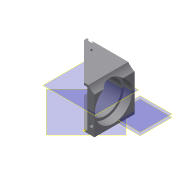
# Autodesk Inventor part: 30_Cube_Insert_Filter_Revolver_Filter_base
Saved by Autodesk Inventor 2019.4 (Build 234330000, 330)
## iProperties
Created: 2021-09-13
Part Number: 30_Cube_Insert_Filter_Revolver_Filter_base
Material: Generic
Document SubType Name: Modeling
Designer: diederichbenedict
Density: 1 g/cm^3
Appearance: Default
Mass: 6.97028 g
Surface Area: 48.8121 cm^2
Volume: 6.97028 cm^3
Author: diederichbenedict
Autodesk Inventor part; units mm, degrees
ref_plane "YZ Plane" through (0, 0, 0) normal (1, 0, 0) x (0, 1, 0)
ref_plane "XZ Plane" through (0, 0, 0) normal (0, 1, 0) x (-1, 0, 0)
ref_plane "XY Plane" through (0, 0, 0) normal (0, 0, 1) x (1, 0, 0)
ref_plane "Work Plane1" through (-34.3358, -34.38, 2.0699) normal (0, -1, 0) x (0.7071068, 0, -0.7071068)
ref_plane "Work Plane4" through (-9.5871, -34.38, 28.2329) normal (0, -1, 0) x (1, 0, 0)
ref_plane "Work Plane3" through (-9.5871, -32.38, 28.2329) normal (0, -1, 0) x (1, 0, 0)
sketch "Sketch1" plane through (-9.5871, -34.38, 28.2329) normal (0, -1, 0) x (1, 0, 0)
  line L0 (-24.2504, -24.2504) -> (-24.2504, -25.6646) construction
  line L1 (-24.2504, -25.6646) -> (0.7071, -0.7071) construction
  line L2 (0.7071, -0.7071) -> (0, 0) construction
  line L3 (-24.2504, -24.2504) -> (0, 0) construction
  line L4 (0.7071, -1.3185) -> (0.7071, -26.3185) construction
  line L5 (0.7071, -1.3185) -> (1.7071, -1.3185) construction
  line L6 (0.7071, -26.3185) -> (1.7071, -26.3185) construction
  line L7 (0.7071, -0.7071) -> (-26.8187, -28.2329)
  line L8 (-26.8187, -28.2329) -> (0.7071, -28.2329)
  line L9 (0.7071, -28.2329) -> (0.7071, -0.7071)
  line L10 (0.7071, -0.7071) -> (5.7071, -0.7071)
  line L11 (5.7071, -0.7071) -> (5.7071, -28.2329)
  line L12 (5.7071, -28.2329) -> (0.7071, -28.2329)
  line L13 (-38.6685, -28.2329) -> (-7.1719, -28.2329) projected
  line L14 (0.7071, -0.7071) -> (5.7071, -0.7071)
  line L15 (5.7071, -0.7071) -> (5.7071, 1.3671)
  line L16 (5.7071, 1.3671) -> (0.7071, 1.3671)
  line L17 (0.7071, 1.3671) -> (0.7071, -0.7071)
  line L18 (2.5336, 1.8671) -> (2.3871, 1.8671) projected
  line L19 (0.7071, -0.7071) -> (0.7071, -28.2329)
  line L20 (0.7071, -28.2329) -> (-26.8187, -28.2329)
  line L21 (-26.8187, -28.2329) -> (0.7071, -0.7071)
  point P0 (9.5871, -28.2329)
  dimension "d1" = 5
  dimension "d2" = 0
  dimension "d3" = 0.5
  constraints: 30 end point, 5 perpendicular, 3 equal length, 3 horizontal, 2 point on line, 2 other
  measures "d1" distance of L9.end L10.end
  measures "d2" distance between parallel lines of L13 L8
  measures "d3" distance between parallel lines of L16 L18
extrude "Extrusion1" add sketch "Sketch1" against normal blind 29 contours L9 L8 L7 | L10 L11 L12 L9
sketch "Sketch2" plane through (-8.88, -34.38, 27.5258) normal (-0.7071068, 0, 0.7071068) x (0.7071068, 0, 0.7071068)
  line L0 (-38.9273, 0) -> (0, 0) projected
  line L1 (0, 0) -> (0, 29) projected
  line L2 (-38.9273, 29) -> (0, 29) projected
  line L3 (-38.9273, 0) -> (-38.9273, 29) projected
  line L4 (-38.9273, 0) -> (-38.9273, 29) projected
  line L5 (-38.9273, 29) -> (0, 29)
  line L6 (0, 29) -> (0, 27.5)
  line L7 (0, 27.5) -> (-38.9273, 27.5)
  line L8 (-38.9273, 27.5) -> (-38.9273, 29)
  line L9 (-38.9273, 0) -> (0, 0)
  line L10 (0, 0) -> (0, 1.5)
  line L11 (0, 1.5) -> (-38.9273, 1.5)
  line L12 (-38.9273, 1.5) -> (-38.9273, 0)
  point P0 (-13.1846, 34.38)
  dimension "d6" = 1.5
  dimension "d7" = 1.5
  constraints: 16 end point, 4 parallel, 2 horizontal, 2 perpendicular, 2 point on line
  measures "d6" distance of L5.end L6.end
  measures "d7" distance of L10.end L9.end
extrude "Extrusion2" add sketch "Sketch2" along normal blind 1.5 contours L3 L11 L1 L0 | L3 L2 L1 L7
sketch "Sketch3" plane through (-3.88, -34.38, 27.5258) normal (1, 0, 0) x (0, 0, -1)
  circle A0 centre (13.1114, 14.5) radius 12.5 projected
  circle A1 centre (13.1114, 14.5) radius 12.8
  point P0 (27.5258, 34.38)
  dimension "d10" = 25.6
  constraints: 1 centre point, 1 coincident
  measures "d10" diameter of A1
extrude "Extrusion3" cut sketch "Sketch3" against normal blind 5.6 contours A0 | A1
sketch "Sketch4" plane through (-3.88, -34.38, 27.5258) normal (1, 0, 0) x (0, 0, -1)
  circle A0 centre (13.1114, 14.5) radius 12.5 projected
  circle A1 centre (13.1114, 14.5) radius 11
  point P0 (27.5258, 34.38)
  dimension "d13" = 22
  constraints: 1 centre point, 1 coincident
  measures "d13" diameter of A1
extrude "Extrusion4" cut sketch "Sketch4" against normal through all contours A1
chamfer "Chamfer1" distance 1.5 angle 45 4 edges at (-9.9407, -6.13, 28.5864) (-9.9407, -33.63, 28.5864) (-37.4664, -6.13, 1.0607) (-37.4664, -33.63, 1.0607)
sketch "Sketch5" plane through (-3.88, -34.38, 0) normal (0, 0, -1) x (-1, 0, 0)
  line L0 (0, 0) -> (32.5258, 0) projected
  line L1 (32.5258, 0) -> (32.5258, 1.5) projected
  line L2 (32.5258, 1.5) -> (32.5258, 27.5) projected
  line L3 (32.5258, 27.5) -> (32.5258, 29) projected
  line L4 (0, 29) -> (32.5258, 29) projected
  line L5 (0, 0) -> (0, 29) projected
  line L6 (30.8258, 1.7) -> (1.7, 1.7)
  line L7 (1.7, 1.7) -> (1.7, 27.3)
  line L8 (1.7, 27.3) -> (30.8258, 27.3)
  line L9 (30.8258, 27.3) -> (30.8258, 1.7)
  circle A0 centre (24.5258, 1.7) radius 1.4
  circle A1 centre (8, 1.7) radius 1.4
  circle A2 centre (8, 27.3) radius 1.4
  circle A3 centre (24.5258, 27.3) radius 1.4
  point P0 (-3.88, 34.38)
  dimension "d19" = 1.7
  dimension "d20" = 2.8
  dimension "d21" = 2.8
  dimension "d22" = 2.8
  dimension "d23" = 2.8
  dimension "d24" = 8
  dimension "d25" = 8
  dimension "d26" = 8
  dimension "d27" = 8
  constraints: 8 end point, 4 centre point, 4 point on line, 3 other
  measures "d19" distance between parallel lines of L0 L6
  measures "d20" diameter of A0
  measures "d21" diameter of A1
  measures "d22" diameter of A2
  measures "d23" diameter of A3
  measures "d24" distance from line of A0.centre L2
  measures "d25" distance from line of A1.centre L5
  measures "d26" distance from line of L5 A2.centre
  measures "d27" distance from line of L2 A3.centre
extrude "Extrusion5" cut sketch "Sketch5" against normal blind 5 contours A0 L6 | L6 A0 | A3 L8 | L8 A3 | A1 L6 | L6 A1 | A2 L8 | L8 A2
sketch "Sketch6" plane through (-3.88, -34.38, 27.5258) normal (0, 0, 1) x (1, 0, 0)
  circle A0 centre (3.88, 34.38) radius 9.7565
  line L0 (0, 0) -> (-32.5258, 0) projected
  line L1 (-32.6288, 1.8364) -> (-30.8098, -0.0697)
  line L2 (-30.8098, -0.0697) -> (-32.6979, -0.0697)
  line L3 (-32.5258, 1.5) -> (-32.5258, 27.5) projected
  line L4 (-32.6979, -0.0697) -> (-32.6288, 1.8364)
  arc A1 (-42.4624, 56.6545) -> (-4.6674, -8.8083) centre (3.9, 39.78) ccw projected
  arc A2 (-37.2068, 12.4952) -> (-23.0987, -1.5152) centre (3.9, 39.78) ccw
  line L5 (-23.0987, -1.5152) -> (-43.2789, -2.9971)
  line L6 (-43.2789, -2.9971) -> (-37.2068, 12.4952)
  point P0 (-25.2852, 0)
  point P1 (-32.5258, 6.5026)
  constraints: 10 end point, 6 point on circle, 2 centre point, 2 point on line, 1 coincident, 1 concentric, 1 perpendicular
extrude "Extrusion6" cut sketch "Sketch6" against normal through all
sketch "Sketch7" plane through (-9.5871, -34.38, 28.2329) normal (0, -1, 0) x (1, 0, 0)
  line L0 (5.7071, -28.2329) -> (-19.5781, -28.2329) projected
  line L1 (5.7071, -0.7071) -> (5.7071, -28.2329) projected
  line L2 (-1.4142, -0.7071) -> (5.7071, -0.7071) projected
  line L3 (-19.5781, -18.871) -> (-1.4142, -0.7071) projected
  line L4 (-1.5524, -3.6738) -> (-0.1382, -5.088)
  line L5 (-0.1382, -5.088) -> (-25.153, -30.1028)
  line L6 (-25.153, -30.1028) -> (-26.5672, -28.6886)
  line L7 (-26.5672, -28.6886) -> (-1.5524, -3.6738)
  line L8 (-19.5781, -18.871) -> (-19.5781, -28.2329) projected
  point P0 (9.5871, -28.2329)
  dimension "d32" = 2
  dimension "d35" = 2
  constraints: 8 end point, 2 parallel, 2 perpendicular
  measures "d32" distance of L4.start L4.end
  measures "d35" distance between parallel lines of L3 L7
extrude "Extrusion7" cut sketch "Sketch7" against normal blind 1.2 contours L8 L7 L4 L5 | L5 L6 L7 L8
ref_plane "Work Plane5" through (-9.5871, -19.88, 28.2329) normal (0, -1, 0) x (1, 0, 0)
mirror "Mirror1" about plane through (-9.5871, -19.88, 28.2329) normal (0, -1, 0) of "Extrusion7"
sketch "Sketch8" plane through (-11.0013, -34.38, 27.5258) normal (0, 0, 1) x (1, 0, 0)
  line L0 (2.8622, 29) -> (0, 29) projected
  line L1 (0, 29) -> (0, 27.5) projected
  line L2 (0, 27.5) -> (2.1213, 27.5) projected
  line L3 (2.1213, 1.5) -> (2.1213, 27.5) projected
  line L4 (2.1213, 1.5) -> (0, 1.5) projected
  line L5 (0, 1.5) -> (0, 0) projected
  line L6 (0, 0) -> (7.1213, 0) projected
  line L7 (7.1213, 0) -> (7.1213, 25.4281) projected
  circle A0 centre (4.732, 5.9773) radius 1.4
  arc A1 (2.8622, 29) -> (7.1213, 25.4281) centre (11.0013, 34.38) ccw projected
  dimension "d36" = 2.8
  constraints: 1 centre point
  measures "d36" diameter of A0
extrude "Extrusion8" cut sketch "Sketch8" against normal up to next contours A0
ref_plane "Work Plane2" through (41.82, -7.88, -4) normal (0, -1, 0) x (1, 0, 0)
body "Solid1"
